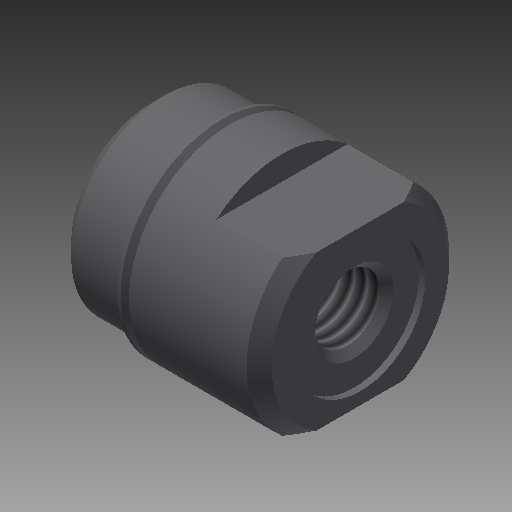
# Autodesk Inventor part: 010000_rear_head
Saved by Autodesk Inventor 2017 (Build 210142000, 142)
## iProperties
Category: PARTsolutions
Company: BIMBA
Created: 2017-01-31
Part Number: 010000_rear_head
Catalog Web Link: www.cadenas.de
Description: Rear Head-Original Line - Standard Air Cylinders
Vendor: BIMBA
Document SubType Name: Modeling
Designer: psAdmin
Manufacturer: BIMBA
Mass: 1.15882 g
Surface Area: 8.95264 cm^2
Volume: 1.15882 cm^3
Density: 1 g/cm^3
Material: Generic
Appearance: PSOLRGB-211-211-211
PSOL_IDENT_0: {$CADENAS_DATA\23d-libs\bimba\bimba\bimba_imperial\bimba_full_line\original_line_cylinders\standard_
PSOL_IDENT_1: air_cylinders\rear_head.prj},227 {VTYP=3D},{NB=010000_rear_head},{LINA=010000_rear_head},{NN=Rear He
PSOL_IDENT_2: ad},{DATE=09.11.2016 07:55:11},{GEOMDATE=30.06.2014 06:34:00},{VERSION=},{LINEID=20},{LINESUBID=-1},
PSOL_IDENT_3: {WBVAR=MNT,ACTING,DER,Q,T1,T2,T3,T4,TRIM,Y,K,MB,CUSH,FBON}  {NB=010000_rear_head},{LINA=010000_rear_
PSOL_IDENT_4: head},{KT=DUMMY},{PN=010000},{BORE=0.43750},{BOREPN=01},{MNT=},{MNTALG='' , 'Front Nose' , 'P' , 'Re
PSOL_IDENT_5: ar Pivot' , 'DX' , 'Double End' , 'BR' , 'Rear Block' , 'BRT' , 'Rear Trunnion'},{ACTING=},{ACTINGAL
PSOL_IDENT_6: G= '' , 'Single Acting' },{DER=},{DERALG= '' , 'Standard' },{Q=},{T1=},{T2=},{T3=},{T4=},{TRIM=0},{Y=
PSOL_IDENT_7: },{K=},{KALG= '', 'without K', 'K', 'with K' },{MB=0},{A1=0.5000},{A1N=0.5000},{A1P=1.1880},{A1B=0.8
PSOL_IDENT_8: 120},{A1S=0.0000},{A2=0.188},{A2N=0.1880},{A3=0.0200},{D1=0.4855},{D1N=0.4855},{D1P=0.7380},{D1B=0.4
PSOL_IDENT_9: 855},{D2=0.4465},{C1=0.0300},{C2=0.0300},{NDM=0.1900},{TAB=UNF},{NDMDP=0.2000},{D3=0.1600},{A4=0.188
PSOL_IDENT_10: 0},{A5=0.3700},{D4=0.0000},{A6=0.0000},{A7=0.5000},{A8=0.1250},{D5=0.4855},{D6=0.1875},{A9=0.6250},{
PSOL_IDENT_11: NDM2=0.4375},{TAB2=UNF},{C11=0.0300},{C22=0.0000},{C33=0.0300},{C44=0.0300},{A10=0.3095},{A11=0.0000
PSOL_IDENT_12: },{NDM3=0.1900},{NDM3N=0.1900},{NDM3B=0.1900},{TAB3=UNF},{TAB3N=UNF},{TAB3B=UNF},{A12=0.5},{A12N=0.5
PSOL_IDENT_13: 000},{A12B=0.4680},{A13=0.9380},{D7=0.1590},{D8=0.4350},{A14=0.0500},{A15=0.0775},{D9=0.3600},{R1=0.
PSOL_IDENT_14: 0315},{X1=0.0000},{X2=0.0000},{CX=0.0000},{CC=0.0000},{CON=0},{S1=0.7500},{DB=0.1562},{X1B=0.2500},{
PSOL_IDENT_15: X2B=0.0620},{A8B=0.1250},{A9B=0.5620},{MODEL=1},{NDM4=0.1640},{TAB4=UNC},{NDM4DP=0.2500},{BC=0.7500}
PSOL_IDENT_16: ,{B1=0.5620},{B2=0.2500},{B3=0.3740},{ON=0},{ON2=1},{G1=0.0000},{G2=0.0000},{G3=0.0000},{G4=0.0000},
PSOL_IDENT_17: {GD=0.0000},{G5=0.0000},{G6=0.0000},{RON=0},{H1=0.0000},{H2=0.0000},{H3=0.0000},{H4=0.0000},{H5=0.00
PSOL_IDENT_18: 00},{H6=0.0000},{F=0.0000},{PNUT=0.0000},{CUSH=0},{CC11=0.000},{CC111=0.0000},{CC22=0.0000},{CC33=0.
PSOL_IDENT_19: 0000},{CC44=0.0000},{CC55=0.0000},{CD1=0.0000},{CD2=0.0000},{CD3=0.0000},{CNDM3=0.0000},{CTAB3=0.000
PSOL_IDENT_20: 0},{OLEN=0.5000},{OD=0.2185},{STDIS=0.0000},{STDIS1=0.0000},{BUSHCON=D-8597},{BUSHL=0.3120},{FBON=0}
PSOL_IDENT_21: ,{LCD=0.0000}
NN: Rear Head
NT: Original Line - Standard Air Cylinders
NB: 010000_rear_head
NBSYN: $PN._rear_head
LINA: 010000_rear_head
PN: 010000
BORE: 0.43750
BOREPN: 01
MNT: Front Nose
MNTALG: '' , 'Front Nose' , 'P' , 'Rear Pivot' , 'DX' , 'Double End' , 'BR' , 'Rear Block' , 'BRT' , 'Rear Trunnion'
ACTING: Single Acting
DER: Standard
Q: Without Side Ported Rear Head
T1: without T1
T2: without T2
T3: without T3
T4: without T4
TRIM: 0
Y: without Pivot Bushing
K: without K
MB: 0
A1N: 0.5000
A1P: 1.1880
A1B: 0.8120
A1S: 0.0000
A2N: 0.1880
A3: 0.0200
D1N: 0.4855
D1P: 0.7380
D1B: 0.4855
D2: 0.4465
C1: 0.0300
C2: 0.0300
TAB: UNF
NDMDP: 0.2000
D3: 0.1600
A4: 0.1880
A5: 0.3700
D4: 0.0000
A6: 0.0000
A7: 0.5000
A8: 0.1250
D5: 0.4855
D6: 0.1875
A9: 0.6250
NDM2: 0.4375
TAB2: UNF
C11: 0.0300
C22: 0.0000
C33: 0.0300
C44: 0.0300
A10: 0.3095
A11: 0.0000
NDM3N: 0.1900
NDM3B: 0.1900
TAB3N: UNF
TAB3B: UNF
A12N: 0.5000
A12B: 0.4680
A13: 0.9380
D7: 0.1590
D8: 0.4350
A14: 0.0500
A15: 0.0775
D9: 0.3600
R1: 0.0315
X1: 0.0000
X2: 0.0000
CX: 0.0000
CC: 0.0000
S1: 0.7500
DB: 0.1562
X1B: 0.2500
X2B: 0.0620
A8B: 0.1250
A9B: 0.5620
NDM4: 0.1640
TAB4: UNC
NDM4DP: 0.2500
BC: 0.7500
B1: 0.5620
B2: 0.2500
B3: 0.3740
G1: 0.0000
G2: 0.0000
G3: 0.0000
G4: 0.0000
GD: 0.0000
G5: 0.0000
G6: 0.0000
H2: 0.0000
H3: 0.0000
F: 0.0000
CUSH: 0
CC111: 0.0000
CC22: 0.0000
CC33: 0.0000
CC44: 0.0000
CC55: 0.0000
CD1: 0.0000
CD2: 0.0000
CD3: 0.0000
CNDM3: 0.0000
CTAB3: 0.0000
OD: 0.2185
STDIS1: 0.0000
BUSHCON: D-8597
BUSHL: 0.3120
FBON: 0
LCD: 0.0000
SUPPLIER: BIMBA
ARTICLENO: 010000_rear_head
BOMINFO: 010000_rear_head
CREATOR: CADENAS GmbH
Title: 010000_rear_head
Author: Cadenas PARTsolutions
Comments: Original Line - Standard Air Cylinders
Autodesk Inventor part; units mm, degrees
sketch "Sketch_1" plane through (0, 0, 0) normal (0, 0, 1) x (1, 0, 0)
  line L0 (12.7, 0) -> (0, 0)
  line L1 (0, 0) -> (0, 4.9085)
  line L2 (0, 4.9085) -> (0.762, 5.6706)
  line L3 (0.762, 5.6706) -> (3.7592, 5.6706)
  line L4 (3.7592, 5.6706) -> (4.2672, 5.1626)
  line L5 (4.2672, 5.1626) -> (4.7752, 5.1626)
  line L6 (4.7752, 5.1626) -> (4.7752, 6.1659)
  line L7 (4.7752, 6.1659) -> (11.938, 6.1659)
  line L8 (11.938, 6.1659) -> (12.7, 5.4039)
  line L9 (12.7, 5.4039) -> (12.7, 0)
  line L10 (12.7, 0) -> (0, 0)
  constraints: 22 end point
revolve "Revolution1" add sketch "Sketch_1" angle 360 about axis through (12.7, 0, 0) along (1, 0, 0)
sketch "Sketch2" plane through (12.7, 0, 0) normal (1, 0, 0) x (0, 0, -1)
  point P0 (0, 0)
hole "Hole1" at (12.7, 0, 0) direction (-1, 0, 0) diameter 7.9248 depth 0.381
sketch "Sketch3" plane through (12.319, 0, 0) normal (1, 0, 0) x (0, 0, -1)
  point P0 (0, 0)
hole "Hole2" at (12.319, 0, 0) direction (-1, 0, 0) diameter 3.9624 depth 12.319 countersink diameter 4.826 countersink angle 90 thread size "10-32 UNF" class "2B" standard "ANSI Unified Screw Threads"
sketch "Sketch_5" plane through (12.7, 0, 0) normal (1, 0, 0) x (0, 0, -1)
  line L0 (-24.6634, -12.3317) -> (24.6634, -12.3317)
  line L1 (24.6634, -12.3317) -> (24.6634, 12.3317)
  line L2 (24.6634, 12.3317) -> (-24.6634, 12.3317)
  line L3 (-24.6634, 12.3317) -> (-24.6634, -12.3317)
  line L4 (-12.3317, -4.699) -> (12.3317, -4.699)
  line L5 (12.3317, -4.699) -> (12.3317, 4.699)
  line L6 (12.3317, 4.699) -> (-12.3317, 4.699)
  line L7 (-12.3317, 4.699) -> (-12.3317, -4.699)
  constraints: 16 end point
extrude "Extrusion1" cut sketch "Sketch_5" against normal blind 4.7752
sketch "Sketch_24" plane through (0, 0, 0) normal (0, 0, 1) x (1, 0, 0)
  line L0 (4.7752, 0) -> (4.2672, 0)
  line L1 (4.0665, 6.1659) -> (4.0665, 6.0817)
  line L2 (4.0665, 6.0817) -> (4.6636, 5.4846)
  arc A0 (4.6636, 5.305) -> (4.6636, 5.4846) centre (4.5738, 5.3948) ccw
  line L3 (4.6636, 5.305) -> (4.5212, 5.1626)
  line L4 (4.5212, 5.1626) -> (4.2672, 5.1626)
  line L5 (4.2672, 5.1626) -> (4.2672, 4.9085)
  line L6 (4.2672, 4.9085) -> (4.7752, 4.9085)
  line L7 (4.7752, 4.9085) -> (4.7752, 5.6603)
  line L8 (4.7752, 5.6603) -> (4.2697, 6.1659)
  line L9 (4.2697, 6.1659) -> (4.0665, 6.1659)
  constraints: 20 end point, 2 point on circle, 1 centre point
revolve "Revolution2" add sketch "Sketch_24" angle 360 about axis through (4.7752, 0, 0) along (1, 0, 0)
ref_plane "cut1_XY" through (12.7, 4.699, 0) normal (1, 0, 0) x (0, 0, -1)
ref_plane "cut1_YZ" through (12.7, 4.699, 0) normal (0, 0, -1) x (0, 1, 0)
ref_plane "cut1_ZX" through (12.7, 4.699, 0) normal (0, 1, 0) x (1, 0, 0)
ref_plane "cut2_XY" through (12.7, -4.699, 0) normal (1, 0, 0) x (0, 0, -1)
ref_plane "cut2_YZ" through (12.7, -4.699, 0) normal (0, 0, -1) x (0, 1, 0)
ref_plane "cut2_ZX" through (12.7, -4.699, 0) normal (0, 1, 0) x (1, 0, 0)
ref_plane "cutf1_XY" through (12.7, 0, 0) normal (0, 0, 1) x (1, 0, 0)
ref_plane "cutf1_YZ" through (12.7, 0, 0) normal (1, 0, 0) x (0, 1, 0)
ref_plane "cutf1_ZX" through (12.7, 0, 0) normal (0, 1, 0) x (0, 0, 1)
ref_plane "cutf2_XY" through (7.9248, 0, 0) normal (0, 0, 1) x (1, 0, 0)
ref_plane "cutf2_YZ" through (7.9248, 0, 0) normal (1, 0, 0) x (0, 1, 0)
ref_plane "cutf2_ZX" through (7.9248, 0, 0) normal (0, 1, 0) x (0, 0, 1)
ref_plane "lovra_XY" through (12.7, 0, 0) normal (1, 0, 0) x (0, 1, 0)
ref_plane "lovra_YZ" through (12.7, 0, 0) normal (0, 1, 0) x (0, 0, 1)
ref_plane "lovra_ZX" through (12.7, 0, 0) normal (0, 0, 1) x (1, 0, 0)
ref_plane "lovra1_XY" through (7.9248, 0, 0) normal (1, 0, 0) x (0, 0, -1)
ref_plane "lovra1_YZ" through (7.9248, 0, 0) normal (0, 0, -1) x (0, 1, 0)
ref_plane "lovra1_ZX" through (7.9248, 0, 0) normal (0, 1, 0) x (1, 0, 0)
ref_plane "lovra2_XY" through (7.9248, 4.699, 0) normal (1, 0, 0) x (0, 0, -1)
ref_plane "lovra2_YZ" through (7.9248, 4.699, 0) normal (0, 0, -1) x (0, 1, 0)
ref_plane "lovra2_ZX" through (7.9248, 4.699, 0) normal (0, 1, 0) x (1, 0, 0)
ref_plane "lovra21_XY" through (0, 0, 5.2705) normal (1, 0, 0) x (0, 0, -1)
ref_plane "lovra21_YZ" through (0, 0, 5.2705) normal (0, 0, -1) x (0, 1, 0)
ref_plane "lovra21_ZX" through (0, 0, 5.2705) normal (0, 1, 0) x (1, 0, 0)
ref_plane "lovra22_XY" through (0, 0, -5.2705) normal (1, 0, 0) x (0, 0, -1)
ref_plane "lovra22_YZ" through (0, 0, -5.2705) normal (0, 0, -1) x (0, 1, 0)
ref_plane "lovra22_ZX" through (0, 0, -5.2705) normal (0, 1, 0) x (1, 0, 0)
ref_plane "lovra3_XY" through (7.9248, -4.699, 0) normal (1, 0, 0) x (0, 0, -1)
ref_plane "lovra3_YZ" through (7.9248, -4.699, 0) normal (0, 0, -1) x (0, 1, 0)
ref_plane "lovra3_ZX" through (7.9248, -4.699, 0) normal (0, 1, 0) x (1, 0, 0)
ref_plane "olen_XY" through (12.7, 0, 0) normal (1, 0, 0) x (0, 0, -1)
ref_plane "olen_YZ" through (12.7, 0, 0) normal (0, 0, -1) x (0, 1, 0)
ref_plane "olen_ZX" through (12.7, 0, 0) normal (0, 1, 0) x (1, 0, 0)
ref_plane "to_mounting_bracket_XY" through (17.4752, 0, 0) normal (1, 0, 0) x (0, 0, -1)
ref_plane "to_mounting_bracket_YZ" through (17.4752, 0, 0) normal (0, 0, -1) x (0, 1, 0)
ref_plane "to_mounting_bracket_ZX" through (17.4752, 0, 0) normal (0, 1, 0) x (1, 0, 0)
ref_plane "to_nut_XY" through (0, 0, 0) normal (1, 0, 0) x (0, 0, -1)
ref_plane "to_nut_YZ" through (0, 0, 0) normal (0, 0, -1) x (0, 1, 0)
ref_plane "to_nut_ZX" through (0, 0, 0) normal (0, 1, 0) x (1, 0, 0)
ref_plane "to_pin_XY" through (23.8252, 0, 0) normal (0, 0, 1) x (1, 0, 0)
ref_plane "to_pin_YZ" through (23.8252, 0, 0) normal (1, 0, 0) x (0, 1, 0)
ref_plane "to_pin_ZX" through (23.8252, 0, 0) normal (0, 1, 0) x (0, 0, 1)
ref_plane "to_screw_XY" through (12.7, 0, 0) normal (0, 1, 0) x (1, 0, 0)
ref_plane "to_screw_YZ" through (12.7, 0, 0) normal (1, 0, 0) x (0, 0, -1)
ref_plane "to_screw_ZX" through (12.7, 0, 0) normal (0, 0, -1) x (0, 1, 0)
ref_plane "to_tube_XY" through (4.2672, 0, 0) normal (1, 0, 0) x (0, 0, -1)
ref_plane "to_tube_YZ" through (4.2672, 0, 0) normal (0, 0, -1) x (0, 1, 0)
ref_plane "to_tube_ZX" through (4.2672, 0, 0) normal (0, 1, 0) x (1, 0, 0)
body "Solid1"
